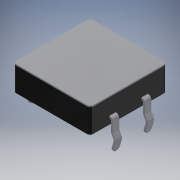
# Autodesk Inventor part: TACT-SWITCH-THT-12X12MM
Saved by Autodesk Inventor 2018.3 (Build 223284000, 284)
## iProperties
Created: 2020-10-19
Part Number: TACT-SWITCH-THT-12X12MM
Material: Genérico
Document SubType Name: Modeling
Designer: laguerre
Density: 8.47 g/cm^3
Appearance: Suave - Negro
Author: laguerre
Autodesk Inventor part; units mm, degrees
ref_plane "YZ Plane" through (0, 0, 0) normal (1, 0, 0) x (0, 1, 0)
ref_plane "XZ Plane" through (0, 0, 0) normal (0, 1, 0) x (-1, 0, 0)
ref_plane "XY Plane" through (0, 0, 0) normal (0, 0, 1) x (1, 0, 0)
sketch "Boceto39" plane through (0, 0, 0) normal (0, 0, 1) x (1, 0, 0)
  line L0 (-5.5, 6) -> (5.5, 6)
  line L1 (6, 5.5) -> (6, -5.5)
  line L2 (5.5, -6) -> (-5.5, -6)
  line L3 (-6, -5.5) -> (-6, 5.5)
  arc A0 (6, 5.5) -> (5.5, 6) centre (5.5, 5.5) ccw
  arc A1 (-5.5, 6) -> (-6, 5.5) centre (-5.5, 5.5) ccw
  arc A2 (-6, -5.5) -> (-5.5, -6) centre (-5.5, -5.5) ccw
  arc A3 (5.5, -6) -> (6, -5.5) centre (5.5, -5.5) ccw
  point P0 (0, 0)
  point P1 (-6, 6)
  point P2 (6, -6)
  point P3 (6, 6)
  point P4 (-6, -6)
  point P5 (0, 6)
  point P6 (6, 0)
  dimension "d373" = 12
  dimension "d376" = 0.5
  constraints: 8 end point, 8 point on circle, 8 point on line, 8 tangent, 4 centre point, 3 equal radius, 2 midpoint, 2 parallel, 2 perpendicular, 1 horizontal, 1 horizontal alignment, 1 vertical alignment
  measures "d373" distance of point (-6, 6) point (6, 6)
  measures "d376" radius of A0
extrude "Extrusión13" add sketch "Boceto39" along normal blind 3.7
sketch "Boceto40" plane through (0, 0, 3.7) normal (0, 0, 1) x (1, 0, 0)
  line L0 (5.5, 6) -> (-5.5, 6) projected
  arc A0 (-5.5, 6) -> (-6, 5.5) centre (-5.5, 5.5) ccw projected
  line L1 (-6, 5.5) -> (-6, -5.5) projected
  arc A1 (-6, -5.5) -> (-5.5, -6) centre (-5.5, -5.5) ccw projected
  line L2 (-5.5, -6) -> (5.5, -6) projected
  arc A2 (5.5, -6) -> (6, -5.5) centre (5.5, -5.5) ccw projected
  line L3 (6, -5.5) -> (6, 5.5) projected
  arc A3 (6, 5.5) -> (5.5, 6) centre (5.5, 5.5) ccw projected
  point P0 (0, 0)
extrude "Extrusión14" add sketch "Boceto40" along normal blind 0.2 separate body
sketch "Boceto43" plane through (0, 0, 0) normal (1, 0, 0) x (0, 1, 0)
  line L0 (0, 0) -> (0, -3.6276) construction
  line L1 (6, 0) -> (6, 3.7) construction
  line L2 (6.05, 1.2) -> (6, 1.2)
  line L3 (5.5, 3.9) -> (-5.5, 3.9) projected
  line L4 (5.5, 0) -> (-5.5, 0) projected
  line L5 (6.55, 0.7) -> (6.55, -0.7482)
  line L6 (6.5752, -0.8453) -> (6.9496, -1.5193)
  line L7 (6.9935, -1.8988) -> (6.5386, -3.5)
  line L8 (6.5386, -3.5) -> (6.25, -3.418)
  line L9 (6.25, -3.418) -> (6.7049, -1.8168)
  line L10 (6.6874, -1.665) -> (6.3129, -0.991)
  line L11 (6.25, -0.7482) -> (6.25, 0.7)
  line L12 (6.05, 0.9) -> (6, 0.9)
  line L13 (6, 0.9) -> (6, 1.2)
  arc A0 (6.25, 0.7) -> (6.05, 0.9) centre (6.05, 0.7) ccw
  arc A1 (6.55, -0.7482) -> (6.5752, -0.8453) centre (6.75, -0.7482) ccw
  arc A2 (6.7049, -1.8168) -> (6.6874, -1.665) centre (6.5126, -1.7622) ccw
  arc A3 (6.55, 0.7) -> (6.05, 1.2) centre (6.05, 0.7) ccw
  arc A4 (6.25, -0.7482) -> (6.3129, -0.991) centre (6.75, -0.7482) ccw
  arc A5 (6.9935, -1.8988) -> (6.9496, -1.5193) centre (6.5126, -1.7622) ccw
  point P0 (6.55, 1.2)
  point P1 (6.55, -0.8)
  point P2 (7.05, -1.7)
  point P3 (6.25, -0.8777)
  dimension "d399" = 2.7
  dimension "d426" = 0.3
  dimension "d427" = 0.3
  dimension "d428" = 0.3
  dimension "d429" = 0.3
  dimension "d430" = 7.05
  dimension "d431" = 6.25
  dimension "d432" = 3.5
  dimension "d433" = 1.8
  dimension "d434" = 2
  dimension "d435" = 0.2
  dimension "d436" = 0.5
  constraints: 22 end point, 12 point on circle, 12 tangent, 10 point on line, 6 centre point, 4 equal radius, 3 perpendicular, 2 parallel, 2 vertical, 1 collinear, 1 vertical alignment
  measures "d399" distance between parallel lines of L2 L3
  measures "d426" distance between parallel lines of L2 L12
  measures "d427" distance between parallel lines of L5 L11
  measures "d428" distance between parallel lines of L6 L10
  measures "d429" distance between parallel lines of L7 L9
  measures "d430" distance from line of point (7.05, -1.7) L0
  measures "d431" distance between parallel lines of L0 L11
  measures "d432" distance from line of L7.end L4
  measures "d433" vertical distance of point (7.05, -1.7) L7.end
  measures "d434" distance from line of L2 point (6.55, -0.8)
  measures "d435" radius of A0
  measures "d436" radius of A3
extrude "Extrusión15" add sketch "Boceto43" along normal mid plane 6 separate body
sketch "Boceto45" plane through (0, 0, 0) normal (1, 0, 0) x (0, 1, 0)
  line L0 (6, 1.2) -> (6.05, 1.2) projected
  line L1 (6, 1.2) -> (7.4698, 1.2)
  line L2 (7.4698, 1.2) -> (7.4698, -3.9971)
  line L3 (7.4698, -3.9971) -> (6, -3.9971)
  line L4 (6, -3.9971) -> (6, 1.2)
  point P0 (0, 0)
  point P1 (3.3, 0.8)
  point P2 (6.05, 1.2)
  constraints: 8 end point, 2 parallel, 1 horizontal, 1 perpendicular, 1 other
extrude "Extrusión17" cut sketch "Boceto45" along normal mid plane 4 bodies 3
fillet "Empalme44" radius 0.5 4 edges at (3, 6.3943, -3.459) (2, 6.3943, -3.459) (-2, 6.3943, -3.459) (-3, 6.3943, -3.459)
mirror "Simetría1" about plane through (0, 0, 0) normal (0, 1, 0) of "Extrusión15", "Extrusión17", "Empalme44" bodies 3
sketch "Boceto46" plane through (0, 0, 3.9) normal (0, 0, 1) x (1, 0, 0)
  line L0 (-2.25, -2.25) -> (2.25, -2.25) construction
  line L1 (2.25, -2.25) -> (2.25, 2.25) construction
  line L2 (2.25, 2.25) -> (-2.25, 2.25) construction
  line L3 (-2.25, 2.25) -> (-2.25, -2.25) construction
  circle A0 centre (-2.25, -2.25) radius 0.4
  circle A1 centre (-2.25, 2.25) radius 0.4
  circle A2 centre (2.25, 2.25) radius 0.4
  circle A3 centre (2.25, -2.25) radius 0.4
  point P0 (0, 0)
  point P1 (0, -2.25)
  point P2 (-2.25, 0)
  dimension "d417" = 0.8
  dimension "d418" = 4.5
  constraints: 8 end point, 4 centre point, 4 coincident, 3 equal radius, 2 midpoint, 2 parallel, 2 perpendicular, 1 horizontal, 1 horizontal alignment, 1 vertical alignment
  measures "d417" diameter of A0
  measures "d418" distance of L1.end L2.end
sketch "Boceto48" plane through (0, 0, 0) normal (0, 1, 0) x (-1, 0, 0)
  line L0 (0, 0) -> (0, 17.1627)
  line L1 (-5.5, 3.9) -> (5.5, 3.9) construction
  line L2 (0, 3.9) -> (-1.75, 3.9)
  line L3 (-1.75, 3.9) -> (-1.6959, 7)
  line L4 (-1.6959, 7) -> (0, 7)
  line L5 (0, 7) -> (0, 3.9)
  line L6 (-5.5, 0) -> (5.5, 0) projected
  line L7 (-1.75, 3.9) -> (-1.75, 4.5675) construction
  dimension "d422" = 7
  dimension "d423" = 3.5
  dimension "d424" = 1
  constraints: 12 end point, 2 perpendicular, 2 point on line, 2 vertical, 1 midpoint
  measures "d422" distance between parallel lines of L6 L4
  measures "d423" diameter of L2.end L0
  measures "d424" angle of L7 L3
